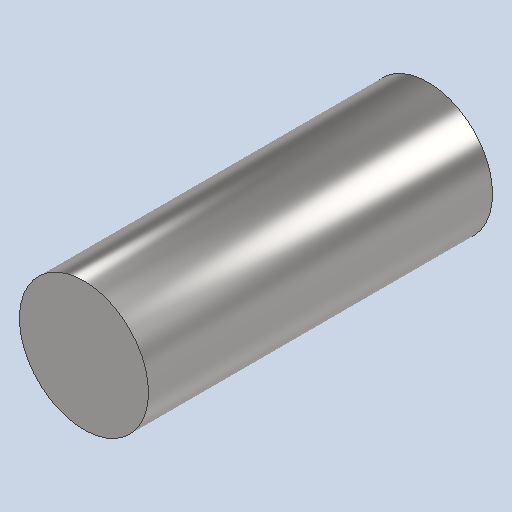
# Autodesk Inventor part: 3mmSchaft_10mm
Saved by Autodesk Inventor 2024 (Build 280153000, 153)
## iProperties
Created: 2022-08-16
Part Number: 3mmSchaft_10mm
Material: Edelstahl
Document SubType Name: Modeling
Designer: alexw
Density: 8 g/cm^3
Appearance: Halbpoliert
Mass: 0.452389 g
Surface Area: 0.895354 cm^2
Volume: 0.0565487 cm^3
Author: alexw
Autodesk Inventor part; units mm, degrees
ref_plane "YZ Plane" through (0, 0, 0) normal (1, 0, 0) x (0, 1, 0)
ref_plane "XZ Plane" through (0, 0, 0) normal (0, 1, 0) x (-1, 0, 0)
ref_plane "XY Plane" through (0, 0, 0) normal (0, 0, 1) x (1, 0, 0)
sketch "Skizze1" plane through (0, 0, 0) normal (0, 0, 1) x (1, 0, 0)
  circle A0 centre (0, 0) radius 1.5
  dimension "d0" = 3
  constraints: 1 centre point, 1 coincident
  measures "d0" diameter of A0
extrude "Extrusion1" add sketch "Skizze1" along normal blind 8
